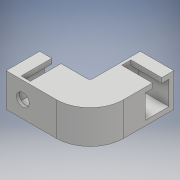
# Autodesk Inventor part: OuterFrame
Saved by Autodesk Inventor 2017 (Build 210142000, 142)
## iProperties
Created: 2017-01-06
Part Number: OuterFrame
Material: Generic
Document SubType Name: Modeling
Designer: kurti
Density: 1 g/cm^3
Appearance: Default
Author: kurti
Autodesk Inventor part; units mm, degrees
ref_plane "YZ Plane" through (0, 0, 0) normal (1, 0, 0) x (0, 1, 0)
ref_plane "XZ Plane" through (0, 0, 0) normal (0, 1, 0) x (-1, 0, 0)
ref_plane "XY Plane" through (0, 0, 0) normal (0, 0, 1) x (1, 0, 0)
sketch "Sketch1" plane through (0, 0, 0) normal (0, 0, 1) x (1, 0, 0)
  line L0 (0, 0) -> (150, 0)
  line L1 (150, 0) -> (150, 45)
  line L2 (90, 60) -> (0, 60)
  line L3 (0, 60) -> (0, 0)
  line L4 (90, 60) -> (90, 150)
  line L5 (90, 150) -> (150, 150)
  line L6 (150, 150) -> (150, 45)
  dimension "d5" = 90
  dimension "d6" = 60
  dimension "d7" = 90
  dimension "d9" = 60
  dimension "d10" = 150
  dimension "d11" = 150
  constraints: 14 end point, 3 parallel, 1 horizontal, 1 perpendicular
  measures "d5" distance of L2.start L2.end
  measures "d6" distance of L2.end L0.start
  measures "d7" distance of L2.start L4.end
  measures "d9" distance of L4.end L5.end
  measures "d10" distance of L0.start L0.end
  measures "d11" distance between parallel lines of L5 L0
extrude "Extrusion1" add sketch "Sketch1" along normal blind 60
sketch "Sketch2" plane through (0, 60, 0) normal (0, 1, 0) x (1, 0, 0)
  line L0 (0, 0) -> (150, 0) construction
  line L1 (0, 0) -> (60, -60) construction
  line L2 (0, 0) -> (84.8528, 0) construction
  line L3 (8.75, -51.25) -> (8.75, -8.75)
  line L4 (8.75, -8.75) -> (51.25, -8.75)
  line L5 (51.25, -8.75) -> (51.25, -51.25)
  line L6 (51.25, -51.25) -> (8.75, -8.75) construction
  line L7 (8.75, -51.25) -> (51.25, -8.75) construction
  line L8 (30, -30) -> (30, -51.25) construction
  line L9 (30, -51.25) -> (21.75, -51.25) construction
  line L10 (30, -51.25) -> (38.25, -51.25) construction
  line L11 (21.75, -51.25) -> (21.75, -60)
  line L12 (0, -60) -> (150, -60) projected
  line L13 (38.25, -51.25) -> (38.25, -60)
  line L14 (21.75, -60) -> (38.25, -60)
  line L15 (51.25, -51.25) -> (38.25, -51.25)
  line L16 (21.75, -51.25) -> (8.75, -51.25)
  dimension "d14" = 84.8528
  dimension "d15" = 45
  dimension "d16" = 42.5
  dimension "d17" = 42.5
  dimension "d32" = 8.25
  dimension "d33" = 8.25
  dimension "d34" = 90
  constraints: 30 end point, 5 parallel, 4 perpendicular, 3 horizontal, 3 midpoint, 2 point on line, 1 equal length, 1 vertical
  measures "d14" distance of L0.start L1.end
  measures "d15" angle of L1 L2
  measures "d16" distance of L3.end L4.end
  measures "d17" distance of L3.start L3.end
  measures "d32" distance of L8.end L9.end
  measures "d33" distance of L10.end L8.end
  measures "d34" angle of L10 L5
extrude "Extrusion2" cut sketch "Sketch2" against normal blind 55
sketch "Sketch4" plane through (150, 0, 0) normal (1, 0, 0) x (0, 0, -1)
  line L0 (0, 150) -> (0, 60) construction
  line L1 (0, 150) -> (-60, 90) construction
  line L2 (0, 150) -> (84.8528, 150) construction
  line L3 (-51.25, 98.75) -> (-8.75, 98.75)
  line L4 (-8.75, 98.75) -> (-8.75, 141.25)
  line L5 (-8.75, 141.25) -> (-51.25, 141.25)
  line L6 (-51.25, 98.75) -> (-8.75, 141.25) construction
  line L7 (-8.75, 98.75) -> (-51.25, 141.25) construction
  line L8 (-30, 120) -> (-60, 120) construction
  line L9 (-60, 120) -> (-60, 128.25)
  line L10 (-60, 0) -> (-60, 150) projected
  line L11 (-60, 128.25) -> (-51.25, 128.25)
  line L12 (-60, 120) -> (-60, 111.75)
  line L13 (-60, 111.75) -> (-51.25, 111.75)
  line L14 (-51.25, 141.25) -> (-51.25, 128.25)
  line L15 (-51.25, 111.75) -> (-51.25, 98.75)
  point P0 (0, 0)
  dimension "d26" = 84.8528
  dimension "d27" = 135
  dimension "d28" = 42.5
  dimension "d29" = 42.5
  dimension "d35" = 8.25
  dimension "d36" = 8.25
  dimension "d37" = 90
  constraints: 28 end point, 6 perpendicular, 3 horizontal, 3 midpoint, 3 parallel, 2 point on line, 1 equal length
  measures "d26" distance of L0.start L1.end
  measures "d27" angle of L1 L2
  measures "d28" distance of L5.end L4.end
  measures "d29" distance of L4.end L3.end
  measures "d35" distance of L8.end L9.end
  measures "d36" distance of L8.end L12.end
  measures "d37" angle of L9 L2
extrude "Extrusion4" cut sketch "Sketch4" against normal blind 55
hole "Hole2" at (30, 5, 30) direction (0, -1, 0) diameter 22.5 end through all
hole "Hole4" at (95, 120, 30) direction (-1, 0, 0) diameter 22.5 end through all
fillet "Fillet1" radius 5 1 edges at (90, 60, 30)
fillet "Fillet2" radius 60 1 edges at (150, 0, 30)
body "Solid1"
